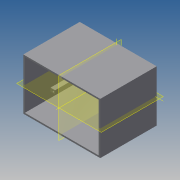
# Autodesk Inventor part: caseBottom
Saved by Autodesk Inventor 2020.4 (Build 244396000, 396)
## iProperties
Created: 2022-05-18
Part Number: caseBottom
Material: Generic
Document SubType Name: Modeling
Designer: Lukas
Density: 1 g/cm^3
Appearance: Default
Author: Lukas
## iProperties of the stored document _3DPrint.ipt
Created: 2022-05-26
Part Number: _3DPrint
Material: Generic
Document SubType Name: Modeling
Designer: Lukas
Density: 1 g/cm^3
Appearance: Default
Author: Lukas
Autodesk Inventor part; units mm, degrees
ref_plane "XY Plane" through (0, 0, 0) normal (0, 0, 1) x (1, 0, 0)
sketch "Sketch1" plane through (0, 0, 0) normal (0, 0, 1) x (1, 0, 0)
  line L0 (0, 70) -> (0, -70) projected
  line L1 (-105, 0) -> (105, 0) projected
  line L2 (-75, 50) -> (75, 50)
  line L3 (75, 50) -> (75, -50)
  line L4 (75, -50) -> (-75, -50)
  line L5 (-75, -50) -> (-75, 50)
  point P0 (0, 50)
  point P1 (75, 0)
  dimension "d1" = 150
  dimension "d2" = 100
  constraints: 8 end point, 2 midpoint, 2 parallel, 2 point on line, 1 horizontal, 1 perpendicular
  measures "d1" distance of L3.end L4.end
  measures "d2" distance of L2.end L3.end
extrude "Extrusion1" add sketch "Sketch1" along normal mid plane 5
sketch "Sketch2" plane through (0, 0, 2.5) normal (0, 0, 1) x (1, 0, 0)
  line L0 (-75, -50) -> (75, -50) construction
  line L1 (75, -50) -> (75, 50) construction
  line L2 (75, 50) -> (-75, 50) construction
  line L3 (-75, 50) -> (-75, -50) construction
  line L4 (-72, 47) -> (72, 47)
  line L5 (72, 47) -> (72, -47)
  line L6 (72, -47) -> (-72, -47)
  line L7 (-72, -47) -> (-72, 47)
  line L8 (-75, 50) -> (75, 50)
  line L9 (75, 50) -> (75, -50)
  line L10 (75, -50) -> (-75, -50)
  line L11 (-75, -50) -> (-75, 50)
  point P0 (0, 0)
  dimension "d5" = 3
  dimension "d6" = 3
  dimension "d7" = 3
  dimension "d8" = 3
  constraints: 16 end point, 4 parallel, 2 horizontal, 2 perpendicular
  measures "d5" distance between parallel lines of L2 L4
  measures "d6" distance between parallel lines of L3 L7
  measures "d7" distance between parallel lines of L1 L5
  measures "d8" distance between parallel lines of L0 L6
extrude "Extrusion2" add sketch "Sketch2" along normal blind 105
sketch "Sketch3" plane through (0, 0, 2.5) normal (0, 0, 1) x (1, 0, 0)
  line L0 (-72, 47) -> (-72, -47) construction
  line L1 (72, 47) -> (-72, 47) construction
  line L2 (-72, -47) -> (-72, 47) construction
  line L3 (-72, 41.69) -> (-63, 41.69)
  line L4 (-63, 41.69) -> (-63, 34.69)
  line L5 (-63, 34.69) -> (-72, 34.69)
  line L6 (-72, 34.69) -> (-72, 41.69)
  line L7 (-72, -29.43) -> (-63, -29.43)
  line L8 (-63, -29.43) -> (-63, -36.43)
  line L9 (-63, -36.43) -> (-72, -36.43)
  line L10 (-72, -36.43) -> (-72, -29.43)
  line L11 (-72, 47) -> (72, 47) construction
  line L12 (45.44, 47) -> (52.44, 47)
  line L13 (52.44, 47) -> (52.44, 35)
  line L14 (52.44, 35) -> (45.44, 35)
  line L15 (45.44, 35) -> (45.44, 47)
  point P0 (0, 0)
  point P1 (-66.63, 38.19)
  point P2 (48.94, 38.19)
  point P3 (-66.63, -32.93)
  dimension "d11" = 5.37
  dimension "d12" = 8.81
  dimension "d13" = 115.57
  dimension "d14" = 8.81
  dimension "d15" = 71.12
  dimension "d16" = 5.37
  dimension "d17" = 7
  dimension "d19" = 9
  dimension "d20" = 7
  dimension "d22" = 9
  dimension "d23" = 7
  dimension "d24" = 12
  dimension "d25" = 3.5
  dimension "d26" = 3.5
  dimension "d67" = 3.5
  constraints: 24 end point, 6 parallel, 3 horizontal, 3 perpendicular, 3 point on line
  measures "d11" distance from line of L0 point (-66.63, 38.19)
  measures "d12" distance from line of L1 point (-66.63, 38.19)
  measures "d13" distance of point (48.94, 38.19) point (-66.63, 38.19)
  measures "d14" distance from line of L1 point (48.94, 38.19)
  measures "d15" distance of point (-66.63, -32.93) point (-66.63, 38.19)
  measures "d16" distance from line of L0 point (-66.63, -32.93)
  measures "d17" distance of L3.end L4.end
  measures "d19" distance between parallel lines of L0 L4
  measures "d20" distance of L7.end L8.end
  measures "d22" distance between parallel lines of L10 L8
  measures "d23" distance of L13.end L14.end
  measures "d24" distance of L12.end L13.end
  measures "d25" distance from line of point (48.94, 38.19) L13
  measures "d26" distance from line of L9 point (-66.63, -32.93)
  measures "d67" distance from line of L3 point (-66.63, 38.19)
extrude "Extrusion3" add sketch "Sketch3" along normal blind 55
sketch "Sketch4" plane through (0, 0, 57.5) normal (0, 0, 1) x (1, 0, 0)
  line L0 (-72, 34.69) -> (-72, 41.69) construction
  line L1 (-72, 47) -> (72, 47) construction
  line L2 (-72, -47) -> (-72, 47) construction
  point P0 (0, 0)
  point P1 (-66.63, 38.19)
  point P2 (-66.63, -32.93)
  point P3 (48.94, 38.19)
  dimension "d29" = 5.37
  dimension "d30" = 8.81
  dimension "d31" = 8.81
  dimension "d32" = 115.57
  dimension "d33" = 71.12
  dimension "d34" = 5.37
  measures "d29" distance from line of L0 point (-66.63, 38.19)
  measures "d30" distance from line of L1 point (-66.63, 38.19)
  measures "d31" distance from line of L1 point (48.94, 38.19)
  measures "d32" distance of point (-66.63, 38.19) point (48.94, 38.19)
  measures "d33" distance of point (-66.63, -32.93) point (-66.63, 38.19)
  measures "d34" distance from line of L2 point (-66.63, -32.93)
hole "Hole1" at (-66.63, 38.19, 57.5) at (-66.63, -32.93, 57.5) at (48.94, 38.19, 57.5) direction (0, 0, -1) diameter 3.6 depth 40 tip angle 118
sketch "Sketch5" plane through (-75, -50, -2.5) normal (-1, 0, 0) x (0, 0, 1)
  line L0 (5, 84.69) -> (60, 84.69) construction
  line L1 (5, 84.69) -> (5, 20.57) construction
  line L2 (5, 82.69) -> (51.8, 82.69)
  line L3 (51.8, 82.69) -> (51.8, 54.49)
  line L4 (51.8, 54.49) -> (5, 54.49)
  line L5 (5, 54.49) -> (5, 82.69)
  point P0 (2.5, 50)
  dimension "d48" = 46.8
  dimension "d49" = 28.2
  dimension "d51" = 2
  constraints: 8 end point, 2 parallel, 1 horizontal, 1 perpendicular, 1 point on line
  measures "d48" distance of L3.end L4.end
  measures "d49" distance of L2.end L3.end
  measures "d51" distance between parallel lines of L0 L2
extrude "Extrusion4" cut sketch "Sketch5" against normal blind 10
sketch "Sketch7" plane through (-75, -50, -2.5) normal (0, -1, 0) x (1, 0, 0)
  line L0 (150, 0) -> (150, 110) construction
  line L1 (150, 0) -> (0, 0) construction
  circle A0 centre (120, 20) radius 8.25
  point P0 (75, 2.5)
  dimension "d52" = 30
  dimension "d53" = 20
  dimension "d54" = 16.5
  constraints: 1 centre point
  measures "d52" distance from line of L0 A0.centre
  measures "d53" distance from line of L1 A0.centre
  measures "d54" diameter of A0
extrude "Extrusion5" cut sketch "Sketch7" against normal blind 10
sketch "Sketch8" plane through (-75, -50, -2.5) normal (0, -1, 0) x (1, 0, 0)
  line L0 (13.4927, 15.961) -> (76.218, 15.961) construction
  line L1 (76.218, 15.961) -> (76.218, 8.9577) construction
  line L2 (76.218, 8.9577) -> (13.4927, 8.9577) construction
  line L3 (13.4927, 8.9577) -> (13.4927, 15.961) construction
  spline S0 degree 2 poles (14.823, 12.2426) (14.4429, 12.2426) (13.9097, 12.4015) (13.6743, 12.5149) knots 0 0 0 1 2 2 2
  line L4 (13.6743, 12.5149) -> (13.6743, 13.0992)
  line L5 (13.6743, 13.0992) -> (13.7083, 13.0992)
  spline S1 degree 2 poles (13.7083, 13.0992) (13.938, 12.8836) (14.5195, 12.6454) (14.7889, 12.6454) knots 0 0 0 1 2 2 2
  spline S2 degree 2 poles (14.7889, 12.6454) (15.1747, 12.6454) (15.5689, 12.9659) (15.5689, 13.2297) knots 0 0 0 1 2 2 2
  spline S3 degree 2 poles (15.5689, 13.2297) (15.5689, 13.4396) (15.3619, 13.7005) (15.1378, 13.7657) knots 0 0 0 1 2 2 2
  spline S4 degree 2 poles (15.1378, 13.7657) (14.9761, 13.8111) (14.7067, 13.8735) (14.5053, 13.9246) knots 0 0 0 1 2 2 2
  spline S5 degree 2 poles (14.5053, 13.9246) (14.3238, 13.9728) (14.0373, 14.1174) (13.9267, 14.2337) knots 0 0 0 1 2 2 2
  spline S6 degree 2 poles (13.9267, 14.2337) (13.8189, 14.35) (13.6998, 14.662) (13.6998, 14.8662) knots 0 0 0 1 2 2 2
  spline S7 degree 2 poles (13.6998, 14.8662) (13.6998, 15.2917) (14.3635, 15.8674) (14.8769, 15.8674) knots 0 0 0 1 2 2 2
  spline S8 degree 2 poles (14.8769, 15.8674) (15.1718, 15.8674) (15.6937, 15.7511) (15.9178, 15.6405) knots 0 0 0 1 2 2 2
  line L6 (15.9178, 15.6405) -> (15.9178, 15.0846)
  line L7 (15.9178, 15.0846) -> (15.8837, 15.0846)
  spline S9 degree 2 poles (15.8837, 15.0846) (15.7164, 15.2378) (15.1945, 15.4647) (14.9081, 15.4647) knots 0 0 0 1 2 2 2
  spline S10 degree 2 poles (14.9081, 15.4647) (14.5847, 15.4647) (14.1848, 15.1612) (14.1848, 14.9144) knots 0 0 0 1 2 2 2
  spline S11 degree 2 poles (14.1848, 14.9144) (14.1848, 14.6932) (14.4202, 14.4294) (14.6414, 14.3699) knots 0 0 0 1 2 2 2
  spline S12 degree 2 poles (14.6414, 14.3699) (14.7889, 14.3302) (15.2172, 14.228) (15.359, 14.1855) knots 0 0 0 1 2 2 2
  spline S13 degree 2 poles (15.359, 14.1855) (15.7192, 14.0749) (16.0539, 13.6296) (16.0539, 13.3034) knots 0 0 0 1 2 2 2
  spline S14 degree 2 poles (16.0539, 13.3034) (16.0539, 13.0964) (15.8866, 12.6993) (15.7363, 12.5603) knots 0 0 0 1 2 2 2
  spline S15 degree 2 poles (15.7363, 12.5603) (15.5689, 12.4071) (15.1435, 12.2426) (14.823, 12.2426) knots 0 0 0 1 2 2 2
  spline S16 degree 2 poles (18.652, 13.6182) (18.652, 12.9545) (18.0138, 12.2313) (17.4806, 12.2313) knots 0 0 0 1 2 2 2
  spline S17 degree 2 poles (17.4806, 12.2313) (16.9332, 12.2313) (16.3064, 12.9772) (16.3064, 13.6182) knots 0 0 0 1 2 2 2
  spline S18 degree 2 poles (16.3064, 13.6182) (16.3064, 14.2763) (16.953, 15.0052) (17.4806, 15.0052) knots 0 0 0 1 2 2 2
  spline S19 degree 2 poles (17.4806, 15.0052) (18.0138, 15.0052) (18.652, 14.2791) (18.652, 13.6182) knots 0 0 0 1 2 2 2
  spline S20 degree 2 poles (18.1953, 13.6182) (18.1953, 14.1288) (17.8238, 14.6251) (17.4806, 14.6251) knots 0 0 0 1 2 2 2
  spline S21 degree 2 poles (17.4806, 14.6251) (17.1374, 14.6251) (16.763, 14.1288) (16.763, 13.6182) knots 0 0 0 1 2 2 2
  spline S22 degree 2 poles (16.763, 13.6182) (16.763, 13.1219) (17.1374, 12.6114) (17.4806, 12.6114) knots 0 0 0 1 2 2 2
  spline S23 degree 2 poles (17.4806, 12.6114) (17.8209, 12.6114) (18.1953, 13.1134) (18.1953, 13.6182) knots 0 0 0 1 2 2 2
  line L8 (19.5568, 12.305) -> (19.1143, 12.305)
  line L9 (19.1143, 12.305) -> (19.1143, 15.961)
  line L10 (19.1143, 15.961) -> (19.5568, 15.961)
  line L11 (19.5568, 15.961) -> (19.5568, 12.305)
  line L12 (22.2257, 12.305) -> (21.7833, 12.305)
  line L13 (21.7833, 12.305) -> (21.7833, 12.5716)
  spline S24 degree 2 poles (21.7833, 12.5716) (21.6811, 12.4866) (21.5308, 12.3731) (21.4287, 12.3249) knots 0 0 0 1 2 2 2
  spline S25 degree 2 poles (21.4287, 12.3249) (21.3351, 12.2795) (21.1337, 12.2313) (21.0004, 12.2313) knots 0 0 0 1 2 2 2
  spline S26 degree 2 poles (21.0004, 12.2313) (20.7849, 12.2313) (20.4218, 12.41) (20.2942, 12.583) knots 0 0 0 1 2 2 2
  spline S27 degree 2 poles (20.2942, 12.583) (20.1666, 12.756) (20.0247, 13.2665) (20.0247, 13.5984) knots 0 0 0 1 2 2 2
  spline S28 degree 2 poles (20.0247, 13.5984) (20.0247, 13.9444) (20.2034, 14.4493) (20.3594, 14.6393) knots 0 0 0 1 2 2 2
  spline S29 degree 2 poles (20.3594, 14.6393) (20.5041, 14.8095) (20.9097, 15.0052) (21.1337, 15.0052) knots 0 0 0 1 2 2 2
  spline S30 degree 2 poles (21.1337, 15.0052) (21.3294, 15.0052) (21.6216, 14.9173) (21.7833, 14.8265) knots 0 0 0 1 2 2 2
  line L14 (21.7833, 14.8265) -> (21.7833, 15.961)
  line L15 (21.7833, 15.961) -> (22.2257, 15.961)
  line L16 (22.2257, 15.961) -> (22.2257, 12.305)
  line L17 (21.7833, 12.9432) -> (21.7833, 14.4606)
  spline S31 degree 2 poles (21.7833, 14.4606) (21.6187, 14.54) (21.3578, 14.5996) (21.2075, 14.5996) knots 0 0 0 1 2 2 2
  spline S32 degree 2 poles (21.2075, 14.5996) (20.8671, 14.5996) (20.4814, 14.0891) (20.4814, 13.6069) knots 0 0 0 1 2 2 2
  spline S33 degree 2 poles (20.4814, 13.6069) (20.4814, 13.1417) (20.7764, 12.6511) (21.1025, 12.6511) knots 0 0 0 1 2 2 2
  spline S34 degree 2 poles (21.1025, 12.6511) (21.2756, 12.6511) (21.6273, 12.8099) (21.7833, 12.9432) knots 0 0 0 1 2 2 2
  spline S35 degree 2 poles (24.0069, 12.2455) (23.3773, 12.2455) (22.6852, 12.9517) (22.6852, 13.6041) knots 0 0 0 1 2 2 2
  spline S36 degree 2 poles (22.6852, 13.6041) (22.6852, 14.2451) (23.3574, 15.0052) (23.8991, 15.0052) knots 0 0 0 1 2 2 2
  spline S37 degree 2 poles (23.8991, 15.0052) (24.1431, 15.0052) (24.5203, 14.8634) (24.6593, 14.7131) knots 0 0 0 1 2 2 2
  spline S38 degree 2 poles (24.6593, 14.7131) (24.8011, 14.5627) (24.9514, 14.1288) (24.9514, 13.8139) knots 0 0 0 1 2 2 2
  line L18 (24.9514, 13.8139) -> (24.9514, 13.5729)
  line L19 (24.9514, 13.5729) -> (23.1333, 13.5729)
  spline S39 degree 2 poles (23.1333, 13.5729) (23.1333, 13.1162) (23.5928, 12.6312) (24.0012, 12.6312) knots 0 0 0 1 2 2 2
  spline S40 degree 2 poles (24.0012, 12.6312) (24.1459, 12.6312) (24.4267, 12.6964) (24.5401, 12.7475) knots 0 0 0 1 2 2 2
  spline S41 degree 2 poles (24.5401, 12.7475) (24.6593, 12.8042) (24.8238, 12.9035) (24.8777, 12.9489) knots 0 0 0 1 2 2 2
  line L20 (24.8777, 12.9489) -> (24.9032, 12.9489)
  line L21 (24.9032, 12.9489) -> (24.9032, 12.4667)
  spline S42 degree 2 poles (24.9032, 12.4667) (24.8266, 12.4355) (24.594, 12.3447) (24.5033, 12.3192) knots 0 0 0 1 2 2 2
  spline S43 degree 2 poles (24.5033, 12.3192) (24.3756, 12.2823) (24.1658, 12.2455) (24.0069, 12.2455) knots 0 0 0 1 2 2 2
  spline S44 degree 2 poles (24.5203, 13.9104) (24.5146, 14.0891) (24.4409, 14.35) (24.37, 14.4379) knots 0 0 0 1 2 2 2
  spline S45 degree 2 poles (24.37, 14.4379) (24.2934, 14.5372) (24.0523, 14.6421) (23.8736, 14.6421) knots 0 0 0 1 2 2 2
  spline S46 degree 2 poles (23.8736, 14.6421) (23.6978, 14.6421) (23.451, 14.5372) (23.3489, 14.4351) knots 0 0 0 1 2 2 2
  spline S47 degree 2 poles (23.3489, 14.4351) (23.2496, 14.3302) (23.1475, 14.0777) (23.1333, 13.9104) knots 0 0 0 1 2 2 2
  line L22 (23.1333, 13.9104) -> (24.5203, 13.9104)
  line L23 (26.7922, 14.4578) -> (26.7695, 14.4578)
  spline S48 degree 2 poles (26.7695, 14.4578) (26.7184, 14.472) (26.6078, 14.4776) (26.5312, 14.4776) knots 0 0 0 1 2 2 2
  spline S49 degree 2 poles (26.5312, 14.4776) (26.3525, 14.4776) (26.0008, 14.3216) (25.842, 14.1685) knots 0 0 0 1 2 2 2
  line L24 (25.842, 14.1685) -> (25.842, 12.305)
  line L25 (25.842, 12.305) -> (25.3995, 12.305)
  line L26 (25.3995, 12.305) -> (25.3995, 14.9315)
  line L27 (25.3995, 14.9315) -> (25.842, 14.9315)
  line L28 (25.842, 14.9315) -> (25.842, 14.54)
  spline S50 degree 2 poles (25.842, 14.54) (26.0831, 14.7556) (26.4433, 14.9315) (26.6135, 14.9315) knots 0 0 0 1 2 2 2
  spline S51 degree 2 poles (26.6135, 14.9315) (26.6816, 14.9315) (26.7496, 14.9258) (26.7922, 14.9173) knots 0 0 0 1 2 2 2
  line L29 (26.7922, 14.9173) -> (26.7922, 14.4578)
  line L30 (27.5863, 12.305) -> (27.1439, 12.305)
  line L31 (27.1439, 12.305) -> (27.1439, 14.9315)
  line L32 (27.1439, 14.9315) -> (27.5863, 14.9315)
  line L33 (27.5863, 14.9315) -> (27.5863, 12.305)
  line L34 (27.6175, 15.3682) -> (27.1155, 15.3682)
  line L35 (27.1155, 15.3682) -> (27.1155, 15.8277)
  line L36 (27.1155, 15.8277) -> (27.6175, 15.8277)
  line L37 (27.6175, 15.8277) -> (27.6175, 15.3682)
  line L38 (30.2978, 12.305) -> (29.8554, 12.305)
  line L39 (29.8554, 12.305) -> (29.8554, 13.8026)
  spline S52 degree 2 poles (29.8554, 13.8026) (29.8554, 13.9841) (29.8213, 14.2961) (29.7703, 14.3897) knots 0 0 0 1 2 2 2
  spline S53 degree 2 poles (29.7703, 14.3897) (29.7164, 14.489) (29.5235, 14.5854) (29.359, 14.5854) knots 0 0 0 1 2 2 2
  spline S54 degree 2 poles (29.359, 14.5854) (29.1945, 14.5854) (28.8457, 14.4096) (28.6783, 14.2678) knots 0 0 0 1 2 2 2
  line L40 (28.6783, 14.2678) -> (28.6783, 12.305)
  line L41 (28.6783, 12.305) -> (28.2358, 12.305)
  line L42 (28.2358, 12.305) -> (28.2358, 14.9315)
  line L43 (28.2358, 14.9315) -> (28.6783, 14.9315)
  line L44 (28.6783, 14.9315) -> (28.6783, 14.6393)
  spline S55 degree 2 poles (28.6783, 14.6393) (28.8769, 14.818) (29.2598, 15.0052) (29.4753, 15.0052) knots 0 0 0 1 2 2 2
  spline S56 degree 2 poles (29.4753, 15.0052) (29.8611, 15.0052) (30.2978, 14.4947) (30.2978, 14.0097) knots 0 0 0 1 2 2 2
  line L45 (30.2978, 14.0097) -> (30.2978, 12.305)
  spline S57 degree 2 poles (31.0126, 11.8853) (31.058, 11.8654) (31.231, 11.803) (31.3416, 11.7775) knots 0 0 0 1 2 2 2
  spline S58 degree 2 poles (31.3416, 11.7775) (31.4636, 11.7463) (31.6706, 11.7094) (31.7926, 11.7094) knots 0 0 0 1 2 2 2
  spline S59 degree 2 poles (31.7926, 11.7094) (31.9968, 11.7094) (32.2804, 11.8172) (32.3598, 11.9136) knots 0 0 0 1 2 2 2
  spline S60 degree 2 poles (32.3598, 11.9136) (32.4364, 12.0101) (32.496, 12.2625) (32.496, 12.4242) knots 0 0 0 1 2 2 2
  line L46 (32.496, 12.4242) -> (32.496, 12.6539)
  spline S61 degree 2 poles (32.496, 12.6539) (32.3173, 12.4979) (31.9741, 12.3504) (31.716, 12.3504) knots 0 0 0 1 2 2 2
  spline S62 degree 2 poles (31.716, 12.3504) (31.2679, 12.3504) (30.7375, 13.0169) (30.7375, 13.6438) knots 0 0 0 1 2 2 2
  spline S63 degree 2 poles (30.7375, 13.6438) (30.7375, 13.9699) (30.9218, 14.4748) (31.075, 14.6535) knots 0 0 0 1 2 2 2
  spline S64 degree 2 poles (31.075, 14.6535) (31.2225, 14.8208) (31.6281, 15.0052) (31.8436, 15.0052) knots 0 0 0 1 2 2 2
  spline S65 degree 2 poles (31.8436, 15.0052) (32.0478, 15.0052) (32.3457, 14.9088) (32.496, 14.8208) knots 0 0 0 1 2 2 2
  line L47 (32.496, 14.8208) -> (32.5215, 14.9315)
  line L48 (32.5215, 14.9315) -> (32.9384, 14.9315)
  line L49 (32.9384, 14.9315) -> (32.9384, 12.6057)
  spline S66 degree 2 poles (32.9384, 12.6057) (32.9384, 11.9363) (32.357, 11.3123) (31.7585, 11.3123) knots 0 0 0 1 2 2 2
  spline S67 degree 2 poles (31.7585, 11.3123) (31.5657, 11.3123) (31.1629, 11.3747) (30.9899, 11.4258) knots 0 0 0 1 2 2 2
  line L50 (30.9899, 11.4258) -> (30.9899, 11.8853)
  line L51 (30.9899, 11.8853) -> (31.0126, 11.8853)
  line L52 (32.496, 13.0169) -> (32.496, 14.4606)
  spline S68 degree 2 poles (32.496, 14.4606) (32.3315, 14.54) (32.0535, 14.6081) (31.9145, 14.6081) knots 0 0 0 1 2 2 2
  spline S69 degree 2 poles (31.9145, 14.6081) (31.5799, 14.6081) (31.1941, 14.1146) (31.1941, 13.6523) knots 0 0 0 1 2 2 2
  spline S70 degree 2 poles (31.1941, 13.6523) (31.1941, 13.2155) (31.4863, 12.7588) (31.8153, 12.7588) knots 0 0 0 1 2 2 2
  spline S71 degree 2 poles (31.8153, 12.7588) (31.9883, 12.7588) (32.3513, 12.895) (32.496, 13.0169) knots 0 0 0 1 2 2 2
  spline S72 degree 2 poles (36.0924, 12.2426) (35.7123, 12.2426) (35.1791, 12.4015) (34.9437, 12.5149) knots 0 0 0 1 2 2 2
  line L53 (34.9437, 12.5149) -> (34.9437, 13.0992)
  line L54 (34.9437, 13.0992) -> (34.9777, 13.0992)
  spline S73 degree 2 poles (34.9777, 13.0992) (35.2075, 12.8836) (35.7889, 12.6454) (36.0584, 12.6454) knots 0 0 0 1 2 2 2
  spline S74 degree 2 poles (36.0584, 12.6454) (36.4441, 12.6454) (36.8384, 12.9659) (36.8384, 13.2297) knots 0 0 0 1 2 2 2
  spline S75 degree 2 poles (36.8384, 13.2297) (36.8384, 13.4396) (36.6313, 13.7005) (36.4072, 13.7657) knots 0 0 0 1 2 2 2
  spline S76 degree 2 poles (36.4072, 13.7657) (36.2456, 13.8111) (35.9761, 13.8735) (35.7747, 13.9246) knots 0 0 0 1 2 2 2
  spline S77 degree 2 poles (35.7747, 13.9246) (35.5932, 13.9728) (35.3068, 14.1174) (35.1961, 14.2337) knots 0 0 0 1 2 2 2
  spline S78 degree 2 poles (35.1961, 14.2337) (35.0884, 14.35) (34.9692, 14.662) (34.9692, 14.8662) knots 0 0 0 1 2 2 2
  spline S79 degree 2 poles (34.9692, 14.8662) (34.9692, 15.2917) (35.6329, 15.8674) (36.1463, 15.8674) knots 0 0 0 1 2 2 2
  spline S80 degree 2 poles (36.1463, 15.8674) (36.4413, 15.8674) (36.9632, 15.7511) (37.1872, 15.6405) knots 0 0 0 1 2 2 2
  line L55 (37.1872, 15.6405) -> (37.1872, 15.0846)
  line L56 (37.1872, 15.0846) -> (37.1532, 15.0846)
  spline S81 degree 2 poles (37.1532, 15.0846) (36.9858, 15.2378) (36.464, 15.4647) (36.1775, 15.4647) knots 0 0 0 1 2 2 2
  spline S82 degree 2 poles (36.1775, 15.4647) (35.8542, 15.4647) (35.4542, 15.1612) (35.4542, 14.9144) knots 0 0 0 1 2 2 2
  spline S83 degree 2 poles (35.4542, 14.9144) (35.4542, 14.6932) (35.6897, 14.4294) (35.9109, 14.3699) knots 0 0 0 1 2 2 2
  spline S84 degree 2 poles (35.9109, 14.3699) (36.0584, 14.3302) (36.4867, 14.228) (36.6285, 14.1855) knots 0 0 0 1 2 2 2
  spline S85 degree 2 poles (36.6285, 14.1855) (36.9887, 14.0749) (37.3234, 13.6296) (37.3234, 13.3034) knots 0 0 0 1 2 2 2
  spline S86 degree 2 poles (37.3234, 13.3034) (37.3234, 13.0964) (37.156, 12.6993) (37.0057, 12.5603) knots 0 0 0 1 2 2 2
  spline S87 degree 2 poles (37.0057, 12.5603) (36.8384, 12.4071) (36.4129, 12.2426) (36.0924, 12.2426) knots 0 0 0 1 2 2 2
  spline S88 degree 2 poles (38.5572, 12.254) (38.1969, 12.254) (37.7914, 12.6652) (37.7914, 13.1105) knots 0 0 0 1 2 2 2
  line L57 (37.7914, 13.1105) -> (37.7914, 14.5656)
  line L58 (37.7914, 14.5656) -> (37.4935, 14.5656)
  line L59 (37.4935, 14.5656) -> (37.4935, 14.9315)
  line L60 (37.4935, 14.9315) -> (37.7914, 14.9315)
  line L61 (37.7914, 14.9315) -> (37.7914, 15.6859)
  line L62 (37.7914, 15.6859) -> (38.2338, 15.6859)
  line L63 (38.2338, 15.6859) -> (38.2338, 14.9315)
  line L64 (38.2338, 14.9315) -> (39.0478, 14.9315)
  line L65 (39.0478, 14.9315) -> (39.0478, 14.5656)
  line L66 (39.0478, 14.5656) -> (38.2338, 14.5656)
  line L67 (38.2338, 14.5656) -> (38.2338, 13.3148)
  spline S89 degree 2 poles (38.2338, 13.3148) (38.2338, 13.1162) (38.248, 12.8978) (38.2962, 12.8042) knots 0 0 0 1 2 2 2
  spline S90 degree 2 poles (38.2962, 12.8042) (38.3359, 12.722) (38.5146, 12.6397) (38.6678, 12.6397) knots 0 0 0 1 2 2 2
  spline S91 degree 2 poles (38.6678, 12.6397) (38.7756, 12.6397) (38.9769, 12.705) (39.0223, 12.7248) knots 0 0 0 1 2 2 2
  line L68 (39.0223, 12.7248) -> (39.0478, 12.7248)
  line L69 (39.0478, 12.7248) -> (39.0478, 12.3277)
  spline S92 degree 2 poles (39.0478, 12.3277) (38.923, 12.2937) (38.6678, 12.254) (38.5572, 12.254) knots 0 0 0 1 2 2 2
  spline S93 degree 2 poles (40.8375, 12.583) (40.7837, 12.5433) (40.6021, 12.4015) (40.517, 12.3589) knots 0 0 0 1 2 2 2
  spline S94 degree 2 poles (40.517, 12.3589) (40.4008, 12.2965) (40.1824, 12.2313) (39.9838, 12.2313) knots 0 0 0 1 2 2 2
  spline S95 degree 2 poles (39.9838, 12.2313) (39.8222, 12.2313) (39.53, 12.3533) (39.4194, 12.4639) knots 0 0 0 1 2 2 2
  spline S96 degree 2 poles (39.4194, 12.4639) (39.3145, 12.5716) (39.1868, 12.8893) (39.1868, 13.0652) knots 0 0 0 1 2 2 2
  spline S97 degree 2 poles (39.1868, 13.0652) (39.1868, 13.3374) (39.4166, 13.7232) (39.6662, 13.8338) knots 0 0 0 1 2 2 2
  spline S98 degree 2 poles (39.6662, 13.8338) (39.8874, 13.9359) (40.4887, 14.0125) (40.8375, 14.0323) knots 0 0 0 1 2 2 2
  line L70 (40.8375, 14.0323) -> (40.8375, 14.1174)
  spline S99 degree 2 poles (40.8375, 14.1174) (40.8375, 14.2706) (40.744, 14.4606) (40.6589, 14.5145) knots 0 0 0 1 2 2 2
  spline S100 degree 2 poles (40.6589, 14.5145) (40.5738, 14.5684) (40.3299, 14.6024) (40.1994, 14.6024) knots 0 0 0 1 2 2 2
  spline S101 degree 2 poles (40.1994, 14.6024) (40.0462, 14.6024) (39.6321, 14.5117) (39.4251, 14.4238) knots 0 0 0 1 2 2 2
  line L71 (39.4251, 14.4238) -> (39.3995, 14.4238)
  line L72 (39.3995, 14.4238) -> (39.3995, 14.8747)
  spline S102 degree 2 poles (39.3995, 14.8747) (39.5215, 14.9088) (39.9781, 14.9938) (40.2022, 14.9938) knots 0 0 0 1 2 2 2
  spline S103 degree 2 poles (40.2022, 14.9938) (40.4745, 14.9938) (40.8461, 14.9088) (40.9935, 14.7981) knots 0 0 0 1 2 2 2
  spline S104 degree 2 poles (40.9935, 14.7981) (41.1382, 14.6904) (41.28, 14.3472) (41.28, 14.1004) knots 0 0 0 1 2 2 2
  line L73 (41.28, 14.1004) -> (41.28, 12.305)
  line L74 (41.28, 12.305) -> (40.8375, 12.305)
  line L75 (40.8375, 12.305) -> (40.8375, 12.583)
  line L76 (40.8375, 12.9517) -> (40.8375, 13.6806)
  spline S105 degree 2 poles (40.8375, 13.6806) (40.6787, 13.6665) (40.1994, 13.6182) (40.0491, 13.5729) knots 0 0 0 1 2 2 2
  spline S106 degree 2 poles (40.0491, 13.5729) (39.8732, 13.519) (39.6435, 13.2949) (39.6435, 13.0964) knots 0 0 0 1 2 2 2
  spline S107 degree 2 poles (39.6435, 13.0964) (39.6435, 12.8695) (39.8987, 12.6397) (40.1427, 12.6397) knots 0 0 0 1 2 2 2
  spline S108 degree 2 poles (40.1427, 12.6397) (40.3497, 12.6397) (40.6901, 12.8184) (40.8375, 12.9517) knots 0 0 0 1 2 2 2
  spline S109 degree 2 poles (42.6953, 12.254) (42.3351, 12.254) (41.9295, 12.6652) (41.9295, 13.1105) knots 0 0 0 1 2 2 2
  line L77 (41.9295, 13.1105) -> (41.9295, 14.5656)
  line L78 (41.9295, 14.5656) -> (41.6317, 14.5656)
  line L79 (41.6317, 14.5656) -> (41.6317, 14.9315)
  line L80 (41.6317, 14.9315) -> (41.9295, 14.9315)
  line L81 (41.9295, 14.9315) -> (41.9295, 15.6859)
  line L82 (41.9295, 15.6859) -> (42.372, 15.6859)
  line L83 (42.372, 15.6859) -> (42.372, 14.9315)
  line L84 (42.372, 14.9315) -> (43.186, 14.9315)
  line L85 (43.186, 14.9315) -> (43.186, 14.5656)
  line L86 (43.186, 14.5656) -> (42.372, 14.5656)
  line L87 (42.372, 14.5656) -> (42.372, 13.3148)
  spline S110 degree 2 poles (42.372, 13.3148) (42.372, 13.1162) (42.3862, 12.8978) (42.4344, 12.8042) knots 0 0 0 1 2 2 2
  spline S111 degree 2 poles (42.4344, 12.8042) (42.4741, 12.722) (42.6528, 12.6397) (42.8059, 12.6397) knots 0 0 0 1 2 2 2
  spline S112 degree 2 poles (42.8059, 12.6397) (42.9137, 12.6397) (43.1151, 12.705) (43.1605, 12.7248) knots 0 0 0 1 2 2 2
  line L88 (43.1605, 12.7248) -> (43.186, 12.7248)
  line L89 (43.186, 12.7248) -> (43.186, 12.3277)
  spline S113 degree 2 poles (43.186, 12.3277) (43.0612, 12.2937) (42.8059, 12.254) (42.6953, 12.254) knots 0 0 0 1 2 2 2
  line L90 (43.9632, 12.305) -> (43.5207, 12.305)
  line L91 (43.5207, 12.305) -> (43.5207, 14.9315)
  line L92 (43.5207, 14.9315) -> (43.9632, 14.9315)
  line L93 (43.9632, 14.9315) -> (43.9632, 12.305)
  line L94 (43.9944, 15.3682) -> (43.4923, 15.3682)
  line L95 (43.4923, 15.3682) -> (43.4923, 15.8277)
  line L96 (43.4923, 15.8277) -> (43.9944, 15.8277)
  line L97 (43.9944, 15.8277) -> (43.9944, 15.3682)
  spline S114 degree 2 poles (46.7711, 13.6182) (46.7711, 12.9545) (46.1329, 12.2313) (45.5997, 12.2313) knots 0 0 0 1 2 2 2
  spline S115 degree 2 poles (45.5997, 12.2313) (45.0523, 12.2313) (44.4255, 12.9772) (44.4255, 13.6182) knots 0 0 0 1 2 2 2
  spline S116 degree 2 poles (44.4255, 13.6182) (44.4255, 14.2763) (45.0722, 15.0052) (45.5997, 15.0052) knots 0 0 0 1 2 2 2
  spline S117 degree 2 poles (45.5997, 15.0052) (46.1329, 15.0052) (46.7711, 14.2791) (46.7711, 13.6182) knots 0 0 0 1 2 2 2
  spline S118 degree 2 poles (46.3145, 13.6182) (46.3145, 14.1288) (45.9429, 14.6251) (45.5997, 14.6251) knots 0 0 0 1 2 2 2
  spline S119 degree 2 poles (45.5997, 14.6251) (45.2565, 14.6251) (44.8821, 14.1288) (44.8821, 13.6182) knots 0 0 0 1 2 2 2
  spline S120 degree 2 poles (44.8821, 13.6182) (44.8821, 13.1219) (45.2565, 12.6114) (45.5997, 12.6114) knots 0 0 0 1 2 2 2
  spline S121 degree 2 poles (45.5997, 12.6114) (45.9401, 12.6114) (46.3145, 13.1134) (46.3145, 13.6182) knots 0 0 0 1 2 2 2
  line L98 (49.2869, 12.305) -> (48.8444, 12.305)
  line L99 (48.8444, 12.305) -> (48.8444, 13.8026)
  spline S122 degree 2 poles (48.8444, 13.8026) (48.8444, 13.9841) (48.8104, 14.2961) (48.7593, 14.3897) knots 0 0 0 1 2 2 2
  spline S123 degree 2 poles (48.7593, 14.3897) (48.7055, 14.489) (48.5126, 14.5854) (48.3481, 14.5854) knots 0 0 0 1 2 2 2
  spline S124 degree 2 poles (48.3481, 14.5854) (48.1836, 14.5854) (47.8347, 14.4096) (47.6674, 14.2678) knots 0 0 0 1 2 2 2
  line L100 (47.6674, 14.2678) -> (47.6674, 12.305)
  line L101 (47.6674, 12.305) -> (47.2249, 12.305)
  line L102 (47.2249, 12.305) -> (47.2249, 14.9315)
  line L103 (47.2249, 14.9315) -> (47.6674, 14.9315)
  line L104 (47.6674, 14.9315) -> (47.6674, 14.6393)
  spline S125 degree 2 poles (47.6674, 14.6393) (47.8659, 14.818) (48.2488, 15.0052) (48.4644, 15.0052) knots 0 0 0 1 2 2 2
  spline S126 degree 2 poles (48.4644, 15.0052) (48.8501, 15.0052) (49.2869, 14.4947) (49.2869, 14.0097) knots 0 0 0 1 2 2 2
  line L105 (49.2869, 14.0097) -> (49.2869, 12.305)
  spline S127 degree 2 poles (53.8193, 13.38) (53.8193, 13.1191) (53.6208, 12.7191) (53.4563, 12.5887) knots 0 0 0 1 2 2 2
  spline S128 degree 2 poles (53.4563, 12.5887) (53.2577, 12.4355) (52.8068, 12.305) (52.4494, 12.305) knots 0 0 0 1 2 2 2
  line L106 (52.4494, 12.305) -> (51.4453, 12.305)
  line L107 (51.4453, 12.305) -> (51.4453, 15.805)
  line L108 (51.4453, 15.805) -> (52.3728, 15.805)
  spline S129 degree 2 poles (52.3728, 15.805) (52.7472, 15.805) (53.1216, 15.7568) (53.2918, 15.6632) knots 0 0 0 1 2 2 2
  spline S130 degree 2 poles (53.2918, 15.6632) (53.4818, 15.5639) (53.6548, 15.2378) (53.6548, 15.0165) knots 0 0 0 1 2 2 2
  spline S131 degree 2 poles (53.6548, 15.0165) (53.6548, 14.7698) (53.3939, 14.3784) (53.1641, 14.2678) knots 0 0 0 1 2 2 2
  line L109 (53.1641, 14.2678) -> (53.1641, 14.2507)
  spline S132 degree 2 poles (53.1641, 14.2507) (53.4761, 14.1656) (53.8193, 13.7147) (53.8193, 13.38) knots 0 0 0 1 2 2 2
  spline S133 degree 2 poles (53.3343, 13.3601) (53.3343, 13.5587) (53.2209, 13.8139) (53.0507, 13.9047) knots 0 0 0 1 2 2 2
  spline S134 degree 2 poles (53.0507, 13.9047) (52.9401, 13.9614) (52.6791, 13.9955) (52.438, 13.9955) knots 0 0 0 1 2 2 2
  line L110 (52.438, 13.9955) -> (51.9105, 13.9955)
  line L111 (51.9105, 13.9955) -> (51.9105, 12.7021)
  line L112 (51.9105, 12.7021) -> (52.2877, 12.7021)
  spline S135 degree 2 poles (52.2877, 12.7021) (52.594, 12.7021) (52.9457, 12.7588) (53.0819, 12.8496) knots 0 0 0 1 2 2 2
  spline S136 degree 2 poles (53.0819, 12.8496) (53.2123, 12.9432) (53.3343, 13.1758) (53.3343, 13.3601) knots 0 0 0 1 2 2 2
  spline S137 degree 2 poles (53.1698, 14.9513) (53.1698, 15.0761) (53.0847, 15.2633) (52.9911, 15.3172) knots 0 0 0 1 2 2 2
  spline S138 degree 2 poles (52.9911, 15.3172) (52.8777, 15.3796) (52.6025, 15.408) (52.3558, 15.408) knots 0 0 0 1 2 2 2
  line L113 (52.3558, 15.408) -> (51.9105, 15.408)
  line L114 (51.9105, 15.408) -> (51.9105, 14.384)
  line L115 (51.9105, 14.384) -> (52.438, 14.384)
  spline S139 degree 2 poles (52.438, 14.384) (52.6564, 14.384) (52.8635, 14.4294) (52.9741, 14.5003) knots 0 0 0 1 2 2 2
  spline S140 degree 2 poles (52.9741, 14.5003) (53.0819, 14.5684) (53.1698, 14.7868) (53.1698, 14.9513) knots 0 0 0 1 2 2 2
  line L116 (56.3096, 14.9315) -> (54.8971, 11.3379)
  line L117 (54.8971, 11.3379) -> (54.4234, 11.3379)
  line L118 (54.4234, 11.3379) -> (54.8943, 12.4327)
  line L119 (54.8943, 12.4327) -> (53.9413, 14.9315)
  line L120 (53.9413, 14.9315) -> (54.4178, 14.9315)
  line L121 (54.4178, 14.9315) -> (55.1354, 12.9857)
  line L122 (55.1354, 12.9857) -> (55.8501, 14.9315)
  line L123 (55.8501, 14.9315) -> (56.3096, 14.9315)
  line L124 (60.2095, 12.305) -> (58.1816, 12.305)
  line L125 (58.1816, 12.305) -> (58.1816, 15.805)
  line L126 (58.1816, 15.805) -> (58.6467, 15.805)
  line L127 (58.6467, 15.805) -> (58.6467, 12.7191)
  line L128 (58.6467, 12.7191) -> (60.2095, 12.7191)
  line L129 (60.2095, 12.7191) -> (60.2095, 12.305)
  line L130 (62.5835, 12.305) -> (62.141, 12.305)
  line L131 (62.141, 12.305) -> (62.141, 12.5943)
  spline S141 degree 2 poles (62.141, 12.5943) (61.9368, 12.4156) (61.5709, 12.2313) (61.344, 12.2313) knots 0 0 0 1 2 2 2
  spline S142 degree 2 poles (61.344, 12.2313) (61.1739, 12.2313) (60.8704, 12.3447) (60.7598, 12.4667) knots 0 0 0 1 2 2 2
  spline S143 degree 2 poles (60.7598, 12.4667) (60.6463, 12.5887) (60.5215, 12.9602) (60.5215, 13.2268) knots 0 0 0 1 2 2 2
  line L132 (60.5215, 13.2268) -> (60.5215, 14.9315)
  line L133 (60.5215, 14.9315) -> (60.964, 14.9315)
  line L134 (60.964, 14.9315) -> (60.964, 13.4339)
  spline S144 degree 2 poles (60.964, 13.4339) (60.964, 13.224) (60.9952, 12.9489) (61.0491, 12.8468) knots 0 0 0 1 2 2 2
  spline S145 degree 2 poles (61.0491, 12.8468) (61.1029, 12.7447) (61.2873, 12.6511) (61.4603, 12.6511) knots 0 0 0 1 2 2 2
  spline S146 degree 2 poles (61.4603, 12.6511) (61.622, 12.6511) (61.9879, 12.8354) (62.141, 12.9687) knots 0 0 0 1 2 2 2
  line L135 (62.141, 12.9687) -> (62.141, 14.9315)
  line L136 (62.141, 14.9315) -> (62.5835, 14.9315)
  line L137 (62.5835, 14.9315) -> (62.5835, 12.305)
  line L138 (65.3999, 12.305) -> (64.8185, 12.305)
  line L139 (64.8185, 12.305) -> (63.8428, 13.5729)
  line L140 (63.8428, 13.5729) -> (63.667, 13.4027)
  line L141 (63.667, 13.4027) -> (63.667, 12.305)
  line L142 (63.667, 12.305) -> (63.2245, 12.305)
  line L143 (63.2245, 12.305) -> (63.2245, 15.961)
  line L144 (63.2245, 15.961) -> (63.667, 15.961)
  line L145 (63.667, 15.961) -> (63.667, 13.8225)
  line L146 (63.667, 13.8225) -> (64.7051, 14.9315)
  line L147 (64.7051, 14.9315) -> (65.2553, 14.9315)
  line L148 (65.2553, 14.9315) -> (64.1775, 13.8338)
  line L149 (64.1775, 13.8338) -> (65.3999, 12.305)
  spline S147 degree 2 poles (67.0847, 12.583) (67.0308, 12.5433) (66.8493, 12.4015) (66.7642, 12.3589) knots 0 0 0 1 2 2 2
  spline S148 degree 2 poles (66.7642, 12.3589) (66.6479, 12.2965) (66.4295, 12.2313) (66.231, 12.2313) knots 0 0 0 1 2 2 2
  spline S149 degree 2 poles (66.231, 12.2313) (66.0693, 12.2313) (65.7772, 12.3533) (65.6666, 12.4639) knots 0 0 0 1 2 2 2
  spline S150 degree 2 poles (65.6666, 12.4639) (65.5616, 12.5716) (65.434, 12.8893) (65.434, 13.0652) knots 0 0 0 1 2 2 2
  spline S151 degree 2 poles (65.434, 13.0652) (65.434, 13.3374) (65.6637, 13.7232) (65.9133, 13.8338) knots 0 0 0 1 2 2 2
  spline S152 degree 2 poles (65.9133, 13.8338) (66.1346, 13.9359) (66.7358, 14.0125) (67.0847, 14.0323) knots 0 0 0 1 2 2 2
  line L150 (67.0847, 14.0323) -> (67.0847, 14.1174)
  spline S153 degree 2 poles (67.0847, 14.1174) (67.0847, 14.2706) (66.9911, 14.4606) (66.906, 14.5145) knots 0 0 0 1 2 2 2
  spline S154 degree 2 poles (66.906, 14.5145) (66.8209, 14.5684) (66.577, 14.6024) (66.4465, 14.6024) knots 0 0 0 1 2 2 2
  spline S155 degree 2 poles (66.4465, 14.6024) (66.2934, 14.6024) (65.8793, 14.5117) (65.6722, 14.4238) knots 0 0 0 1 2 2 2
  line L151 (65.6722, 14.4238) -> (65.6467, 14.4238)
  line L152 (65.6467, 14.4238) -> (65.6467, 14.8747)
  spline S156 degree 2 poles (65.6467, 14.8747) (65.7687, 14.9088) (66.2253, 14.9938) (66.4494, 14.9938) knots 0 0 0 1 2 2 2
  spline S157 degree 2 poles (66.4494, 14.9938) (66.7217, 14.9938) (67.0932, 14.9088) (67.2407, 14.7981) knots 0 0 0 1 2 2 2
  spline S158 degree 2 poles (67.2407, 14.7981) (67.3854, 14.6904) (67.5272, 14.3472) (67.5272, 14.1004) knots 0 0 0 1 2 2 2
  line L153 (67.5272, 14.1004) -> (67.5272, 12.305)
  line L154 (67.5272, 12.305) -> (67.0847, 12.305)
  line L155 (67.0847, 12.305) -> (67.0847, 12.583)
  line L156 (67.0847, 12.9517) -> (67.0847, 13.6806)
  spline S159 degree 2 poles (67.0847, 13.6806) (66.9259, 13.6665) (66.4465, 13.6182) (66.2962, 13.5729) knots 0 0 0 1 2 2 2
  spline S160 degree 2 poles (66.2962, 13.5729) (66.1204, 13.519) (65.8906, 13.2949) (65.8906, 13.0964) knots 0 0 0 1 2 2 2
  spline S161 degree 2 poles (65.8906, 13.0964) (65.8906, 12.8695) (66.1459, 12.6397) (66.3898, 12.6397) knots 0 0 0 1 2 2 2
  spline S162 degree 2 poles (66.3898, 12.6397) (66.5969, 12.6397) (66.9372, 12.8184) (67.0847, 12.9517) knots 0 0 0 1 2 2 2
  spline S163 degree 2 poles (68.8574, 12.2426) (68.5936, 12.2426) (68.137, 12.3844) (67.9867, 12.4639) knots 0 0 0 1 2 2 2
  line L157 (67.9867, 12.4639) -> (67.9867, 12.9602)
  line L158 (67.9867, 12.9602) -> (68.0093, 12.9602)
  spline S164 degree 2 poles (68.0093, 12.9602) (68.0661, 12.9148) (68.2192, 12.8071) (68.3469, 12.7475) knots 0 0 0 1 2 2 2
  spline S165 degree 2 poles (68.3469, 12.7475) (68.4575, 12.6936) (68.7298, 12.6142) (68.8744, 12.6142) knots 0 0 0 1 2 2 2
  spline S166 degree 2 poles (68.8744, 12.6142) (68.9794, 12.6142) (69.2205, 12.6624) (69.2772, 12.7021) knots 0 0 0 1 2 2 2
  spline S167 degree 2 poles (69.2772, 12.7021) (69.3594, 12.756) (69.4332, 12.878) (69.4332, 13.0028) knots 0 0 0 1 2 2 2
  spline S168 degree 2 poles (69.4332, 13.0028) (69.4332, 13.1588) (69.263, 13.3204) (69.0446, 13.3743) knots 0 0 0 1 2 2 2
  spline S169 degree 2 poles (69.0446, 13.3743) (68.9595, 13.3942) (68.6872, 13.4509) (68.5709, 13.4821) knots 0 0 0 1 2 2 2
  spline S170 degree 2 poles (68.5709, 13.4821) (68.2703, 13.57) (67.998, 13.9331) (67.998, 14.1912) knots 0 0 0 1 2 2 2
  spline S171 degree 2 poles (67.998, 14.1912) (67.998, 14.5485) (68.5341, 14.9938) (68.9765, 14.9938) knots 0 0 0 1 2 2 2
  spline S172 degree 2 poles (68.9765, 14.9938) (69.1949, 14.9938) (69.6374, 14.8861) (69.7877, 14.8038) knots 0 0 0 1 2 2 2
  line L159 (69.7877, 14.8038) -> (69.7877, 14.3302)
  line L160 (69.7877, 14.3302) -> (69.765, 14.3302)
  spline S173 degree 2 poles (69.765, 14.3302) (69.5948, 14.4663) (69.1807, 14.6223) (68.968, 14.6223) knots 0 0 0 1 2 2 2
  spline S174 degree 2 poles (68.968, 14.6223) (68.7496, 14.6223) (68.449, 14.4379) (68.449, 14.2536) knots 0 0 0 1 2 2 2
  spline S175 degree 2 poles (68.449, 14.2536) (68.449, 14.0862) (68.6277, 13.9246) (68.8262, 13.8735) knots 0 0 0 1 2 2 2
  spline S176 degree 2 poles (68.8262, 13.8735) (68.9226, 13.848) (69.1666, 13.7969) (69.2999, 13.7657) knots 0 0 0 1 2 2 2
  spline S177 degree 2 poles (69.2999, 13.7657) (69.5892, 13.692) (69.8841, 13.3545) (69.8841, 13.0623) knots 0 0 0 1 2 2 2
  spline S178 degree 2 poles (69.8841, 13.0623) (69.8841, 12.8921) (69.7508, 12.5915) (69.6204, 12.4809) knots 0 0 0 1 2 2 2
  spline S179 degree 2 poles (69.6204, 12.4809) (69.4814, 12.3646) (69.1269, 12.2426) (68.8574, 12.2426) knots 0 0 0 1 2 2 2
  point P0 (75, 2.5)
  constraints: 2 other
extrude "Extrusion6" cut sketch "Sketch8" against normal blind 1
sketch "Sketch9" plane through (0, 0, 2.5) normal (0, 0, 1) x (1, 0, 0)
  line L0 (-72, -47) -> (72, -47) construction
  line L1 (72, -47) -> (72, 47) construction
  circle A0 centre (-8, 0) radius 15
  point P0 (0, 0)
  dimension "d59" = 30
  dimension "d60" = 80
  dimension "d61" = 47
  constraints: 1 centre point
  measures "d59" diameter of A0
  measures "d60" distance from line of L1 A0.centre
  measures "d61" distance from line of L0 A0.centre
extrude "Extrusion7" add sketch "Sketch9" along normal blind 40
sketch "Sketch11" plane through (0, 0, 2.5) normal (0, 0, 1) x (1, 0, 0)
  line L0 (-72, 47) -> (72, 47) construction
  line L1 (72, 47) -> (65, 47)
  line L2 (65, 47) -> (65, 40)
  line L3 (65, 40) -> (72, 40)
  line L4 (72, 40) -> (72, 47)
  line L5 (72, 47) -> (72, -47) construction
  line L6 (72, -47) -> (65, -47)
  line L7 (65, -47) -> (65, -40)
  line L8 (65, -40) -> (72, -40)
  line L9 (72, -40) -> (72, -47)
  point P0 (0, 0)
  dimension "d68" = 7
  dimension "d69" = 7
  dimension "d70" = 7
  dimension "d71" = 7
  constraints: 16 end point, 4 parallel, 2 horizontal, 2 perpendicular
  measures "d68" distance of L3.end L2.end
  measures "d69" distance of L2.end L1.end
  measures "d70" distance of L7.end L8.end
  measures "d71" distance of L6.end L7.end
extrude "Extrusion8" add sketch "Sketch11" along normal blind 95
sketch "Sketch12" plane through (0, 0, 107.5) normal (0, 0, 1) x (1, 0, 0)
  line L0 (-75, -50) -> (75, -50) construction
  line L1 (75, -50) -> (75, 50) construction
  line L2 (75, 50) -> (-75, 50) construction
  point P0 (0, 0)
  point P1 (69.5, 44.5)
  point P2 (69.5, -44.5)
  dimension "d74" = 5.5
  dimension "d75" = 5.5
  dimension "d76" = 5.5
  dimension "d77" = 5.5
  measures "d74" distance from line of L1 point (69.5, 44.5)
  measures "d75" distance from line of L2 point (69.5, 44.5)
  measures "d76" distance from line of L1 point (69.5, -44.5)
  measures "d77" distance from line of L0 point (69.5, -44.5)
hole "Hole2" at (69.5, 44.5, 107.5) at (69.5, -44.5, 107.5) direction (0, 0, -1) diameter 3.6 depth 40 tip angle 118
body "Solid1"
